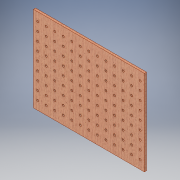
# Autodesk Inventor part: copy_stand_base
Saved by Autodesk Inventor 2019 (Build 230136000, 136)
## iProperties
Created: 2018-12-01
Part Number: copy_stand_base
Material: Generic
Document SubType Name: Modeling
Designer: caleb
Density: 1 g/cm^3
Appearance: White Oak - Natural Medium Gloss
Author: caleb
Autodesk Inventor part; units mm, degrees
ref_plane "YZ Plane" through (0, 0, 0) normal (1, 0, 0) x (0, 1, 0)
ref_plane "XZ Plane" through (0, 0, 0) normal (0, 1, 0) x (-1, 0, 0)
ref_plane "XY Plane" through (0, 0, 0) normal (0, 0, 1) x (1, 0, 0)
sketch "Sketch1" plane through (0, 0, 0) normal (0, 0, 1) x (1, 0, 0)
  line L0 (-165.1, -127) -> (165.1, -127)
  line L1 (165.1, -127) -> (165.1, 127)
  line L2 (165.1, 127) -> (-165.1, 127)
  line L3 (-165.1, 127) -> (-165.1, -127)
  line L4 (-165.1, -127) -> (165.1, 127) construction
  line L5 (165.1, -127) -> (-165.1, 127) construction
  point P0 (0, 0)
  dimension "d0" = 254
  dimension "d1" = 330.2
  constraints: 12 end point, 2 midpoint, 2 parallel, 1 horizontal, 1 perpendicular
  measures "d0" distance of L0.end L1.end
  measures "d1" distance of L0.start L0.end
extrude "Extrusion1" add sketch "Sketch1" along normal blind 6.35
sketch "Sketch3" plane through (0, 0, 6.35) normal (0, 0, 1) x (1, 0, 0)
  point P0 (0, 0)
  point P1 (0, 0)
  dimension "d4" = 215.9
  dimension "d5" = 60
  dimension "d6" = 68.6924
  dimension "d7" = 152.4
  constraints: 1 coincident
hole "Hole1" at (0, 0, 6.35) direction (0, 0, -1) diameter 6.35 end through all
pattern_linear "Rectangular Pattern1" count 9 spacing 25.4 along (0, -1, 0) count 13 spacing 25.4 along (-1, 0, 0) of "Hole1" first direction both ways yes second direction both ways yes
body "Solid1"
